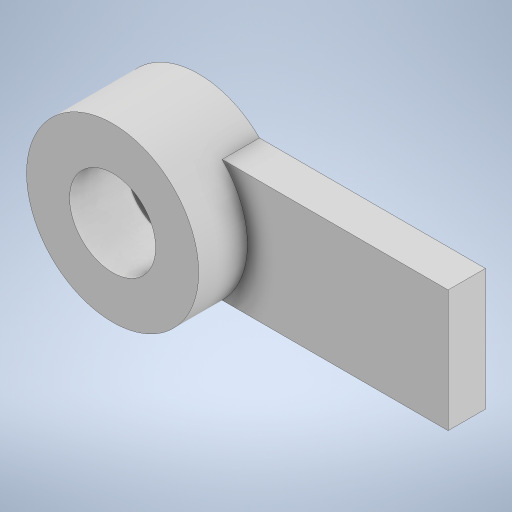
# Autodesk Inventor part: rod_end_fixation
Saved by Autodesk Inventor 2024 (Build 280153000, 153)
## iProperties
Created: 2024-02-23
Part Number: rod_end_fixation
Material: Generic
Document SubType Name: Modeling
Designer: clbri
Density: 1 g/cm^3
Appearance: Default
Author: clbri
Autodesk Inventor part; units mm, degrees
ref_plane "YZ Plane" through (0, 0, 0) normal (1, 0, 0) x (0, 1, 0)
ref_plane "XZ Plane" through (0, 0, 0) normal (0, 1, 0) x (-1, 0, 0)
ref_plane "XY Plane" through (0, 0, 0) normal (0, 0, 1) x (1, 0, 0)
sketch "Sketch1" plane through (0, 0, 0) normal (0, 0, 1) x (1, 0, 0)
  circle A0 centre (0, 0) radius 6
  dimension "d1" = 12
  constraints: 1 centre point
  measures "d1" diameter of A0
extrude "Extrusion1" add sketch "Sketch1" along normal blind 6
sketch "Sketch2" plane through (0, 0, 6) normal (0, 0, 1) x (1, 0, 0)
  circle A0 centre (0, 0) radius 3
  dimension "d4" = 6
  constraints: 1 centre point, 1 coincident
  measures "d4" diameter of A0
extrude "Extrusion2" cut sketch "Sketch2" against normal blind 4
sketch "Sketch3" plane through (0, 0, 0) normal (0, 0, -1) x (-1, 0, 0)
  line L0 (0, 4.25) -> (-20, 4.25)
  line L1 (-20, 4.25) -> (-20, -4.25)
  line L2 (-20, -4.25) -> (0, -4.25)
  circle A0 centre (0, 0) radius 3
  line L3 (0, -4.25) -> (0, -3)
  line L4 (0, 3) -> (0, 4.25)
  dimension "d7" = 20
  dimension "d8" = 8.5
  dimension "d9" = 4.25
  dimension "d10" = 6
  constraints: 10 end point, 3 parallel, 2 point on circle, 1 centre point, 1 coincident, 1 horizontal, 1 perpendicular
  measures "d7" distance of L2.end L1.end
  measures "d8" distance of L1.end L0.end
  measures "d9" distance from line of point (0, 0) L0
  measures "d10" diameter of A0
extrude "Extrusion3" add sketch "Sketch3" against normal blind 2.6 contours L4 A0 L3 L2 L1 L0
body "Solid1"
